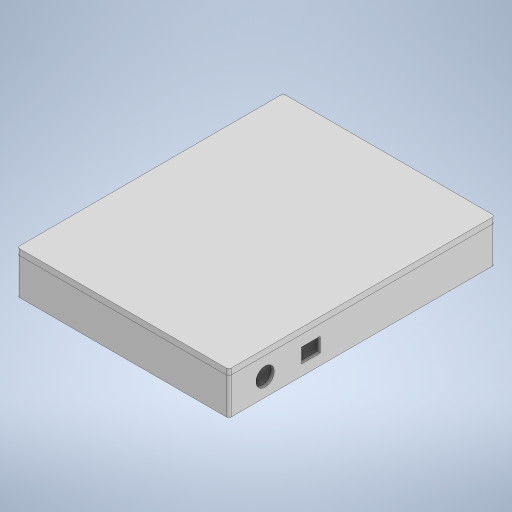
# Autodesk Inventor part: Enclosure-Draft-1
Saved by Autodesk Inventor 2023 (Build 270158000, 158)
## iProperties
Created: 2024-03-22
Part Number: Enclosure-Draft-1
Material: Generic
Document SubType Name: Modeling
Designer: ongyu
Density: 1 g/cm^3
Appearance: Default
Author: ongyu
Autodesk Inventor part; units mm, degrees
ref_plane "YZ Plane" through (0, 0, 0) normal (1, 0, 0) x (0, 1, 0)
ref_plane "XZ Plane" through (0, 0, 0) normal (0, 1, 0) x (-1, 0, 0)
ref_plane "XY Plane" through (0, 0, 0) normal (0, 0, 1) x (1, 0, 0)
sketch "Sketch1" plane through (0, 0, 0) normal (0, 1, 0) x (-1, 0, 0)
  line L0 (87.5, -110) -> (-87.5, -110)
  line L1 (-87.5, -110) -> (-87.5, 110)
  line L2 (-87.5, 110) -> (87.5, 110)
  line L3 (87.5, 110) -> (87.5, -110)
  line L4 (0, -154) -> (0, 154) projected
  line L5 (-122.5, 0) -> (122.5, 0) projected
  point P0 (0, 0)
  dimension "d0" = 175
  dimension "d1" = 220
  dimension "d2" = 87.5
  dimension "d3" = 110
  constraints: 8 end point, 2 parallel, 1 horizontal, 1 perpendicular
  measures "d0" distance between parallel lines of L3 L1
  measures "d1" distance between parallel lines of L2 L0
  measures "d2" distance between parallel lines of L4 L1
  measures "d3" distance between parallel lines of L5 L0
extrude "Extrusion1" add sketch "Sketch1" along normal blind 5
sketch "Sketch2" plane through (0, 0, 0) normal (0, -1, 0) x (1, 0, 0)
  line L0 (87.5, 110) -> (87.5, -110) projected
  line L1 (-87.5, 110) -> (87.5, 110) projected
  line L2 (-87.5, -110) -> (-87.5, 110) projected
  line L3 (87.5, -110) -> (-87.5, -110) projected
  point P0 (0, 0)
extrude "Extrusion2" add sketch "Sketch2" along normal blind 30 separate body
fillet "Fillet1" radius 2 8 edges at (-87.5, 2.5, -110) (-87.5, 2.5, 110) (87.5, 2.5, 110) (87.5, 2.5, -110) (-87.5, -15, -110) (-87.5, -15, 110) (87.5, -15, 110) (87.5, -15, -110)
sketch "Sketch3" plane through (87.5, 0, 108) normal (1, 0, 0) x (0, 0, -1)
  circle A0 centre (28, -15) radius 7.5
  line L0 (216, -30) -> (0, -30) projected
  line L1 (0, 0) -> (216, 0) projected
  line L2 (-2, 0) -> (-2, -30) projected
  line L3 (58, -9) -> (73.5, -9)
  line L4 (73.5, -9) -> (73.5, -21)
  line L5 (73.5, -21) -> (58, -21)
  line L6 (58, -21) -> (58, -9)
  point P0 (108, 0)
  dimension "d9" = 15
  dimension "d10" = 30
  dimension "d11" = 15
  dimension "d12" = 30
  dimension "d13" = 15.5
  dimension "d14" = 12
  dimension "d15" = 9
  dimension "d16" = 30
  constraints: 8 end point, 2 parallel, 1 centre point, 1 horizontal, 1 perpendicular
  measures "d9" diameter of A0
  measures "d10" distance between parallel lines of L0 L1
  measures "d11" distance from line of A0.centre L1
  measures "d12" distance from line of L2 A0.centre
  measures "d13" distance between parallel lines of L6 L4
  measures "d14" distance between parallel lines of L5 L3
  measures "d15" distance between parallel lines of L3 L1
  measures "d16" distance from line of A0.centre L6
extrude "Extrusion3" cut sketch "Sketch3" against normal blind 2.5 bodies 2
shell "Shell1" thickness 1 removed faces 2 at (85, -17.1538, 77.7864) at (85, -17, 44.8333) bodies 2
equation "\"d2\" = 0.5 * d0"
equation "\"d3\" = 0.5 * d1"
equation "\"d11\" = 0.5 * d10"
equation "\"d15\" = -0.5 * d14 + 0.5 * d10"
body "Solid1"
body "Solid2"
